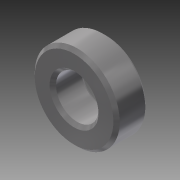
# Autodesk Inventor part: BearingRadialBall4x8x3
Saved by Autodesk Inventor 2015 SP1 (Build 190203100, 203)
## iProperties
Category: Hardware
Created: 2014-12-01
Part Number: BearingRadialBall4x8x3
Material: Steel, Alloy
Document SubType Name: Modeling
Designer: Jack
Density: 7.73 g/cm^3
Appearance: Semi-Polished
Mass: 0.848015 g
Surface Area: 1.75245 cm^2
Volume: 0.109704 cm^3
Vendor: Hobbyking / eBay
Stock Number: B674ZZ
Author: Jack
Title: Bearing Radial Ball 4x8x3
Comments: Wonky bearing size that should be changed.
Autodesk Inventor part; units mm, degrees
ref_plane "YZ Plane" through (0, 0, 0) normal (1, 0, 0) x (0, 1, 0)
ref_plane "XZ Plane" through (0, 0, 0) normal (0, 1, 0) x (-1, 0, 0)
ref_plane "XY Plane" through (0, 0, 0) normal (0, 0, 1) x (1, 0, 0)
sketch "Sketch1" plane through (0, 0, 0) normal (0, 1, 0) x (-1, 0, 0)
  circle A0 centre (0, 0) radius 2
  circle A1 centre (0, 0) radius 4
  dimension "d0" = 4
  dimension "d1" = 8
  constraints: 2 centre point, 2 coincident
  measures "d0" diameter of A0
  measures "d1" diameter of A1
extrude "Extrusion1" add sketch "Sketch1" along normal blind 3
chamfer "Chamfer1" distance 0.3 angle 45 4 edges at (4, 3, 0) (4, 0, 0) (2, 3, 0) (2, 0, 0)
body "Solid1"
